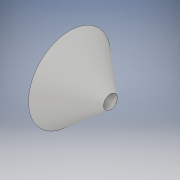
# Autodesk Inventor part: mocowania_magnesów
Saved by Autodesk Inventor 2017 SP1 (Build 210196100, 196)
## iProperties
Part Number: mocowania_magnesów
Material: Ogólny
Document SubType Name: Modeling
Designer: Bartosz
Density: 1 g/cm^3
Appearance: Domyślna
Author: Bartosz
Autodesk Inventor part; units mm, degrees
ref_plane "YZ Plane" through (0, 0, 0) normal (1, 0, 0) x (0, 1, 0)
ref_plane "XZ Plane" through (0, 0, 0) normal (0, 1, 0) x (-1, 0, 0)
ref_plane "XY Plane" through (0, 0, 0) normal (0, 0, 1) x (1, 0, 0)
sketch "Szkic1" plane through (0, 0, 0) normal (0, 0, 1) x (1, 0, 0)
  line L0 (0, 0) -> (3, 0)
  line L1 (3, 0) -> (3, 0.5)
  line L2 (0, 0) -> (0, 3)
  line L3 (0, 3) -> (3, 0.5)
  dimension "d3" = 3
  dimension "d4" = 0.5
  constraints: 8 end point, 1 horizontal, 1 perpendicular, 1 vertical
  measures "d3" distance of L0.start L0.end
  measures "d4" distance of L0.end L1.end
revolve "Obrót1" add sketch "Szkic1" angle 360 about axis through (0, 0, 0) along (1, 0, 0)
hole "Otwór1" at (3, -0.0058, 0) direction (-1, 0, 0) diameter 1 end through all
